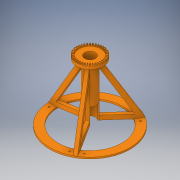
# Autodesk Inventor part: Base
Saved by Autodesk Inventor 2018 (Build 220112000, 112)
## iProperties
Created: 2017-08-26
Part Number: Base
Material: Generic
Document SubType Name: Modeling
Designer: ToreDenStore
Density: 1 g/cm^3
Appearance: Default
Author: ToreDenStore
Autodesk Inventor part; units mm, degrees
ref_plane "YZ Plane" through (0, 0, 0) normal (1, 0, 0) x (0, 1, 0)
sketch "Sketch2" plane through (0, 0, 0) normal (0, 1, 0) x (-1, 0, 0)
  circle A0 centre (0, 0) radius 75
  circle A1 centre (0, 0) radius 60
  dimension "d0" = 150
  dimension "d1" = 15
  constraints: 2 centre point, 2 coincident
  measures "d0" diameter of A0
  measures "d1" radial gap between concentric circles of A1 A0
extrude "Extrusion1" add sketch "Sketch2" along normal blind 3
ref_plane "Work Plane1" through (0, 10, 0) normal (0, -1, 0) x (1, 0, 0)
sketch "Sketch3" plane through (0, 10, 0) normal (0, -1, 0) x (1, 0, 0)
  circle A0 centre (0, 0) radius 10
  circle A1 centre (0, 0) radius 12
  dimension "d5" = 20
  dimension "d6" = 2
  constraints: 2 centre point, 2 coincident
  measures "d5" diameter of A0
  measures "d6" radial gap between concentric circles of A1 A0
extrude "Extrusion2" add sketch "Sketch3" against normal blind 100
ref_plane "Work Plane2" through (0, 0, 3) normal (0, 0, 1) x (1, 0, 0)
sketch "Sketch5" plane through (0, 0, 3) normal (0, 0, 1) x (1, 0, 0)
  line L0 (75, 3) -> (-75, 3) projected
  line L1 (12, 110) -> (-12, 110) projected
  line L2 (-75, 3) -> (-12, 110)
  line L3 (-12, 10) -> (-12, 110) projected
  line L4 (-12, 10) -> (-60, 3)
  line L5 (-12, 94.2325) -> (-61.046, 10.9321)
  line L6 (-61.046, 10.9321) -> (-12, 18.0846)
  point P0 (0, 0)
  dimension "d14" = 15
  dimension "d15" = 8
  dimension "d16" = 8
  constraints: 8 end point, 3 point on line, 2 parallel
  measures "d14" distance of L0.end L4.end
  measures "d15" distance between parallel lines of L5 L2
  measures "d16" distance between parallel lines of L6 L4
extrude "Extrusion3" add sketch "Sketch5" against normal blind 6 contours L0 L2 L3 L5 L6 L4
sketch "Sketch6" plane through (0, 110, 0) normal (0, 1, 0) x (1, 0, 0)
  line L0 (-12, 0) -> (-12, 3) projected
  circle A0 centre (0, 0) radius 12 projected
  line L1 (-12, -3) -> (-12, 0) projected
  line L2 (-12, 3) -> (-60, 3) projected
  line L3 (-12, 3) -> (-11.619, 3)
  line L4 (-12, -3) -> (-11.619, -3)
  constraints: 4 end point, 2 point on circle, 1 collinear, 1 parallel
extrude "Extrusion4" add sketch "Sketch6" against normal blind 100 contours L0 L3 A0 | A0 L4 L1
pattern_circular "Circular Pattern1" count 3 over 360 about axis through (0, 10, 0) along (0, 1, 0) of "Extrusion3", "Extrusion4"
sketch "Sketch7" plane through (0, 10, 0) normal (0, -1, 0) x (1, 0, 0)
  arc A0 (8.4076, -8.5623) -> (8.4076, 8.5623) centre (0, 0) ccw projected
  circle A1 centre (0, 0) radius 10 projected
  line L0 (8.4076, 8.5623) -> (7.0063, 7.1353)
  line L1 (7.0063, -7.1353) -> (8.4076, -8.5623)
  arc A2 (8.4076, -8.5623) -> (8.4076, 8.5623) centre (0, 0) ccw projected
  line L2 (7.0063, 7.1353) -> (2.1815, 2.2216) construction
  line L3 (0, 0) -> (7.0063, -7.1353) construction
  line L4 (8.5981, -8.8923) -> (32.5981, -50.4615) projected
  line L5 (2.1815, 2.2216) -> (0, 0) construction
  dimension "d27" = 0
  dimension "d28" = 0
  constraints: 10 end point, 4 point on circle, 3 collinear, 1 point on line
  measures "d27" distance of A0.start L1.end
  measures "d28" distance of A0.end L0.start
extrude "Extrusion5" cut sketch "Sketch7" against normal blind 30 contours L1 A1 L0 A0
sketch "Sketch8" plane through (0, 110, 0) normal (0, 1, 0) x (1, 0, 0)
  circle A0 centre (0, 0) radius 10 projected
  circle A1 centre (0, 0) radius 25
  dimension "d31" = 50
  constraints: 1 centre point, 1 coincident
  measures "d31" diameter of A1
extrude "Extrusion6" add sketch "Sketch8" along normal blind 5
sketch "Sketch9" plane through (0, 115, 0) normal (0, 1, 0) x (1, 0, 0)
  circle A0 centre (0, 0) radius 25 projected
  line L0 (0, 0) -> (-0.8245, 20.9838) construction
  line L1 (0.9815, 24.9807) -> (0.8245, 20.9838)
  line L2 (0, 25) -> (0, 0) construction
  arc A1 (0.8245, 20.9838) -> (-0.8245, 20.9838) centre (0, 0) ccw
  arc A2 (-0.8245, 20.9838) -> (0.8245, 20.9838) centre (0, 0) ccw construction
  line L3 (0.8245, 20.9838) -> (0, 0) construction
  line L4 (-0.8245, 20.9838) -> (-0.9815, 24.9807)
  dimension "d34" = 4.5
  dimension "d36" = 4
  dimension "d37" = 2.25
  constraints: 10 end point, 7 point on circle, 2 centre point, 2 collinear, 1 coincident, 1 vertical
  measures "d34" angle of L1 L0
  measures "d36" radial gap between concentric circles of A0 A1
  measures "d37" angle of L1 L2
extrude "Extrusion7" add sketch "Sketch9" along normal blind 3 contours L1 A1 L4 A0 picked at (-0.0916, 23.6646)
chamfer "Chamfer1" distance 2 angle 20 1 edges at (0.903, 118, -22.9823) measured on face at (0.903, 117.5, -22.9823)
chamfer "Chamfer2" distance 2 angle 20 1 edges at (-0.903, 118, -22.9823) measured on face at (-0.903, 117.5, -22.9823)
pattern_circular "Circular Pattern2" count 40 over 360 about axis through (0, 10, 0) along (0, 1, 0) of "Extrusion7", "Chamfer1", "Chamfer2"
sketch "Sketch10" plane through (0, 3, 0) normal (0, 1, 0) x (1, 0, 0)
  circle A0 centre (0, 0) radius 60 projected
  line L0 (105, 0) -> (-105, 0) projected
  circle A1 centre (0, 0) radius 67.5
  point P0 (-66.7551, 10)
  dimension "d51" = 10
  dimension "d52" = 7.5
  constraints: 1 coincident, 3 other
  measures "d51" distance from line of L0 point (-66.755, 10)
hole "Hole1" at (-66.7551, 3, -10) direction (0, -1, 0) diameter 3 end through all
mirror "Mirror1" about plane through (0, 0, 0) normal (0, 0, 1) of "Hole1"
pattern_circular "Circular Pattern3" count 3 over 360 about axis through (0, 10, 0) along (0, 1, 0) of "Hole1", "Mirror1"
